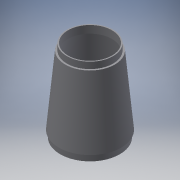
# Autodesk Inventor part: Transición
Saved by Autodesk Inventor 2019.4 (Build 234330000, 330)
## iProperties
Created: 2022-01-21
Part Number: Transición
Material: Generic
Document SubType Name: Modeling
Designer: juand
Density: 1 g/cm^3
Appearance: Default
Author: juand
Autodesk Inventor part; units mm, degrees
ref_plane "YZ Plane" through (0, 0, 0) normal (1, 0, 0) x (0, 1, 0)
ref_plane "XZ Plane" through (0, 0, 0) normal (0, 1, 0) x (-1, 0, 0)
ref_plane "XY Plane" through (0, 0, 0) normal (0, 0, 1) x (1, 0, 0)
sketch "Sketch2" plane through (0, 0, 0) normal (0, 0, 1) x (1, 0, 0)
  line L0 (25.15, 75) -> (27, 75)
  line L1 (25.15, 75) -> (25.15, 82)
  line L2 (25.15, 82) -> (23.95, 82)
  line L3 (23.95, 82) -> (23.95, 73.8)
  line L4 (23.95, 73.8) -> (25.964, 73.8)
  line L5 (27, 75) -> (25.15, 75)
  line L6 (34, 0) -> (27, 75)
  line L7 (32.5, 0) -> (32.5, -7)
  line L8 (32.5, -7) -> (31.3, -7)
  line L9 (31.3, -7) -> (31.3, 1.2)
  line L10 (31.3, 1.2) -> (32.6828, 1.2)
  line L11 (32.6828, 1.2) -> (25.9068, 73.8)
  line L12 (34, 0) -> (32.5, 0)
  line L13 (0, -24.8) -> (0, 99.8) projected
  point P0 (0, 0)
  dimension "d20" = 7
  dimension "d21" = 1.2
  dimension "d23" = 1.2
  dimension "d31" = 34
  dimension "d33" = 7
  dimension "d34" = 1.2
  dimension "d36" = 1.2
  dimension "d37" = 75
  dimension "d38" = 27
  dimension "d39" = 25.15
  dimension "d40" = 32.5
  constraints: 26 end point, 4 horizontal, 2 parallel, 2 perpendicular, 1 point on line, 1 vertical
  measures "d20" distance of L0.start L1.end
  measures "d21" distance of L1.end L2.end
  measures "d23" distance between parallel lines of L4 L0
  measures "d31" distance of point (0, 0) L6.start
  measures "d33" distance of L7.start L7.end
  measures "d34" distance of L7.end L8.end
  measures "d36" distance between parallel lines of L6 L11
  measures "d37" vertical distance of L6.start L0.end
  measures "d38" horizontal distance of point (0, 0) L0.end
  measures "d39" horizontal distance of point (0, 0) L0.start
  measures "d40" distance of point (0, 0) L7.start
revolve "Revolution3" add sketch "Sketch2" angle 360 about axis through (0, -10, 0) along (0, 1, 0)
body "Solid3"
